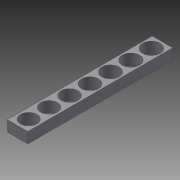
# Autodesk Inventor part: hole_test
Saved by Autodesk Inventor 2015 (Build 190159000, 159)
## iProperties
Created: 2015-01-04
Part Number: hole_test
Material: Generic
Document SubType Name: Modeling
Designer: Drew
Density: 1 g/cm^3
Appearance: Default
Author: Drew
Autodesk Inventor part; units mm, degrees
ref_plane "YZ Plane" through (0, 0, 0) normal (1, 0, 0) x (0, 1, 0)
ref_plane "XZ Plane" through (0, 0, 0) normal (0, 1, 0) x (-1, 0, 0)
ref_plane "XY Plane" through (0, 0, 0) normal (0, 0, 1) x (1, 0, 0)
sketch "Sketch1" plane through (0, 0, 0) normal (0, 1, 0) x (-1, 0, 0)
  line L0 (-6, -42.5) -> (6, -42.5)
  line L1 (6, -42.5) -> (6, 42.5)
  line L2 (6, 42.5) -> (-6, 42.5)
  line L3 (-6, 42.5) -> (-6, -42.5)
  line L4 (-6, -42.5) -> (6, 42.5) construction
  line L5 (6, -42.5) -> (-6, 42.5) construction
  point P0 (0, 0)
  point P1 (0, 0)
  dimension "d6" = 12
  dimension "d7" = 85
  constraints: 12 end point, 4 midpoint, 2 parallel, 1 horizontal, 1 perpendicular
  measures "d6" distance of L1.end L2.end
  measures "d7" distance of L0.end L1.end
extrude "Extrusion1" add sketch "Sketch1" along normal blind 6.35
sketch "Sketch2" plane through (0, 6.35, 0) normal (0, 1, 0) x (1, 0, 0)
  circle A0 centre (0, -36) radius 4.85
  line L0 (0, -55.0438) -> (0, 59.6363)
  circle A1 centre (0, -24) radius 4.9
  circle A2 centre (0, -12) radius 4.95
  circle A3 centre (0, 0) radius 5
  circle A4 centre (0, 12) radius 5.05
  circle A5 centre (0, 24) radius 5.1
  circle A6 centre (0, 36) radius 5.15
  point P0 (0, 0)
  dimension "d10" = 9.7
  dimension "d11" = 9.8
  dimension "d12" = 9.9
  dimension "d13" = 10
  dimension "d14" = 10.1
  dimension "d15" = 10.2
  dimension "d16" = 12
  dimension "d17" = 12
  dimension "d18" = 12
  dimension "d19" = 12
  dimension "d20" = 12
  dimension "d21" = 10.3
  dimension "d22" = 12
  constraints: 7 centre point, 1 coincident, 10 other
  measures "d10" diameter of A0
  measures "d11" diameter of A1
  measures "d12" diameter of A2
  measures "d13" diameter of A3
  measures "d14" diameter of A4
  measures "d15" diameter of A5
  measures "d16" distance of A1.centre A0.centre
  measures "d17" distance of A2.centre A1.centre
  measures "d18" distance of point (0, 0) A2.centre
  measures "d19" distance of point (0, 0) A4.centre
  measures "d20" distance of A4.centre A5.centre
  measures "d21" diameter of A6
  measures "d22" distance of A5.centre A6.centre
extrude "Extrusion2" cut sketch "Sketch2" against normal up to surface (6.35 mm away)
equation "\"d17\" = d16"
equation "\"d18\" = d16"
equation "\"d19\" = d16"
equation "\"d20\" = d16"
equation "\"d22\" = d16"
body "Solid1"
